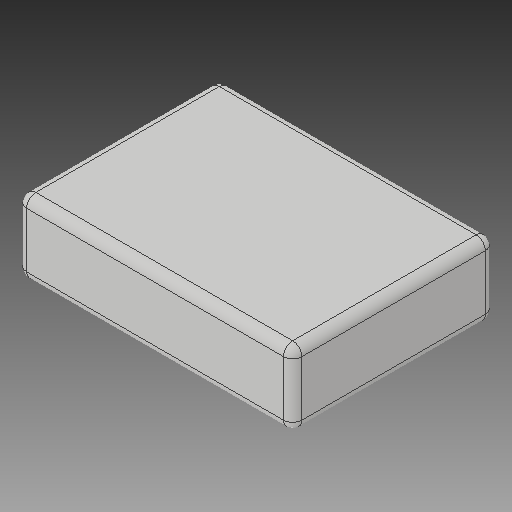
# Autodesk Inventor part: AM-3205 AP radio
Saved by Autodesk Inventor 2019.4 (Build 234330000, 330)
## iProperties
Created: 2017-12-16
Part Number: AM-3205 AP radio
Material: Generic
Document SubType Name: Modeling
Designer: TODD D MILLER
Density: 1 g/cm^3
Appearance: Default
Author: TODD D MILLER
Autodesk Inventor part; units mm, degrees
ref_plane "YZ Plane" through (0, 0, 0) normal (1, 0, 0) x (0, 1, 0)
ref_plane "XZ Plane" through (0, 0, 0) normal (0, 1, 0) x (-1, 0, 0)
ref_plane "XY Plane" through (0, 0, 0) normal (0, 0, 1) x (1, 0, 0)
sketch "Sketch1" plane through (0, 0, 0) normal (0, 1, 0) x (-1, 0, 0)
  line L0 (47.625, 34.925) -> (-47.625, 34.925)
  line L1 (-47.625, 34.925) -> (-47.625, -34.925)
  line L2 (-47.625, -34.925) -> (47.625, -34.925)
  line L3 (47.625, -34.925) -> (47.625, 34.925)
  line L4 (47.625, 34.925) -> (-47.625, -34.925) construction
  line L5 (-47.625, 34.925) -> (47.625, -34.925) construction
  point P0 (0, 0)
  dimension "d0" = 95.25
  dimension "d1" = 69.85
  constraints: 12 end point, 2 midpoint, 2 parallel, 1 horizontal, 1 perpendicular
  measures "d0" distance of L2.end L1.end
  measures "d1" distance of L1.end L0.end
extrude "Extrusion1" add sketch "Sketch1" along normal blind 25.4
fillet "Fillet1" radius 3.175 12 edges at (-47.625, 25.4, 0) (0, 25.4, -34.925) (47.625, 12.7, -34.925) (47.625, 25.4, 0) (47.625, 12.7, 34.925) (0, 25.4, 34.925) (-47.625, 12.7, 34.925) (0, 0, 34.925) (-47.625, 0, 0) (0, 0, -34.925) (-47.625, 12.7, -34.925) (47.625, 0, 0)
body "Solid1"
